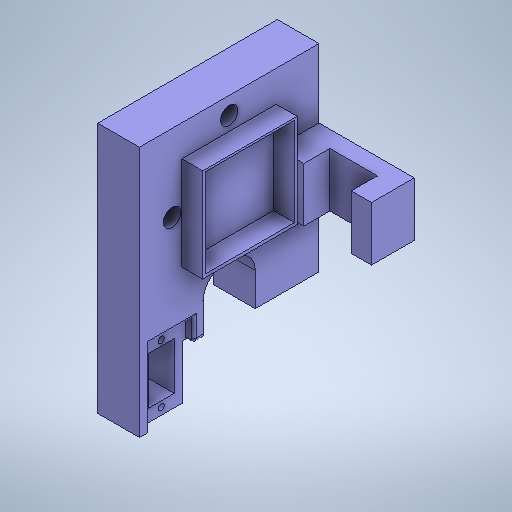
# Autodesk Inventor part: HolderWStepper
Saved by Autodesk Inventor 2025.1 (Build 291241000, 241)
## iProperties
Created: 2024-10-19
Part Number: HolderWStepper
Material: Generic
Document SubType Name: Modeling
Designer: 13156
Density: 1 g/cm^3
Appearance: Default
Author: 13156
Autodesk Inventor part; units mm, degrees
ref_plane "YZ Plane" through (0, 0, 0) normal (1, 0, 0) x (0, 1, 0)
ref_plane "XZ Plane" through (0, 0, 0) normal (0, 1, 0) x (-1, 0, 0)
ref_plane "XY Plane" through (0, 0, 0) normal (0, 0, 1) x (1, 0, 0)
sketch "Sketch1" plane through (0, 0, 0) normal (1, 0, 0) x (0, 1, 0)
  line L0 (-4.3, 12.5) -> (-12.5, 12.5)
  line L1 (-4.3, -12.5) -> (-12.5, -12.5)
  line L2 (-12.5, 12.5) -> (-12.5, 18.5)
  line L3 (-12.5, 18.5) -> (23.4392, 18.5)
  line L4 (23.4392, 18.5) -> (23.4392, -18.5)
  line L5 (23.4392, -18.5) -> (-12.5, -18.5)
  line L6 (-12.5, -18.5) -> (-12.5, -12.5)
  line L7 (23.4392, 0) -> (13.4392, 0) construction
  line L8 (13.4392, 0) -> (0, 0) construction
  line L9 (10.7392, -7.25) -> (10.7392, 0) construction
  line L10 (10.7392, 0) -> (10.7392, 7.25) construction
  line L11 (-4.3, 12.5) -> (13.4392, 12.5)
  line L12 (13.4392, 12.5) -> (13.4392, -12.5)
  line L13 (13.4392, -12.5) -> (-4.3, -12.5)
  point P0 (-8.4, 12.5)
  dimension "d0" = 8.2
  dimension "d1" = 25
  dimension "d2" = 12.5
  dimension "d7" = 8.2
  dimension "d8" = 12.5
  dimension "d9" = 12.5
  dimension "d14" = 6
  dimension "d15" = 6
  dimension "d16" = 37
  dimension "d29" = 10
  dimension "d88" = 2.7
  dimension "d90" = 14.5
  dimension "d91" = 23.4392
  dimension "d92" = 15.0392
  constraints: 28 end point, 5 perpendicular, 4 horizontal, 3 point on line, 2 midpoint, 1 collinear, 1 vertical
  measures "d0" distance of L0.start L0.end
  measures "d1" distance between parallel lines of L1 L0
  measures "d2" vertical distance of point (-8.4, 12.5) L8.end
  measures "d7" distance of L1.start L1.end
  measures "d8" vertical distance of L1.start L8.end
  measures "d9" horizontal distance of L1.end L8.end
  measures "d14" distance of L0.end L2.end
  measures "d15" distance of L5.end L1.end
  measures "d16" distance of L3.end L4.end
  measures "d29" distance of L7.start L7.end
  measures "d88" distance from line of L9 L7.end
  measures "d90" distance of L10.end L9.start
  measures "d91" distance of L7.start L8.end
  measures "d92" horizontal distance of L1.start L9.start
extrude "Extrusion1" add sketch "Sketch1" along normal blind 20
sketch "Sketch2" plane through (0, 23.4392, 18.5) normal (0, 1, 0) x (1, 0, 0)
  line L0 (0, 31) -> (0, 37) projected
  line L1 (0, 37) -> (70, 37)
  line L2 (70, 37) -> (70, 0.0995)
  line L3 (70, 0.0995) -> (0, 0.0995)
  line L4 (0, 0.0995) -> (0, 37)
  line L5 (20, 37) -> (20, 0) projected
  point P0 (0, 18.5)
  point P1 (70, 18.5498)
  dimension "d19" = 50
  constraints: 8 end point, 2 parallel, 1 horizontal, 1 midpoint, 1 perpendicular
  measures "d19" distance from line of L5 point (70, 18.55)
extrude "Extrusion2" add sketch "Sketch2" along normal blind 10
sketch "Sketch3" plane through (0, 23.4392, 18.5) normal (0, -1, 0) x (1, 0, 0)
  line L0 (110.5, -8.5498) -> (110.5, -28.5498)
  line L1 (110.5, -28.5498) -> (70, -28.5498)
  line L2 (70, -28.5498) -> (70, -8.5498)
  line L3 (70, -0.0995) -> (70, -37) projected
  line L4 (110.5, -8.5498) -> (119.5, -8.5498)
  line L5 (119.5, -8.5498) -> (119.5, -37)
  line L6 (119.5, -37) -> (70, -37)
  line L7 (70, -37) -> (0, -37) projected
  line L8 (70, -37) -> (59, -37)
  line L9 (59, -37) -> (59, -8.5498)
  line L10 (59, -8.5498) -> (70, -8.5498)
  point P0 (0, -18.5)
  point P1 (70, -18.5498)
  point P2 (70, -18.5498)
  point P3 (110.5, -18.5498)
  dimension "d22" = 20
  dimension "d23" = 20
  dimension "d24" = 0
  dimension "d25" = 40.5
  dimension "d26" = 9
  dimension "d30" = 11
  constraints: 18 end point, 4 perpendicular, 3 midpoint, 2 point on line, 2 vertical, 1 horizontal
  measures "d22" distance of L0.start L0.end
  measures "d23" distance of L1.end L2.end
  measures "d24" distance of point (70, -18.55) point (70, -18.55)
  measures "d25" distance from line of L2 point (110.5, -18.55)
  measures "d26" distance between parallel lines of L0 L5
  measures "d30" distance between parallel lines of L9 L2
extrude "Extrusion3" add sketch "Sketch3" along normal blind 9.5 and the other way blind 10
sketch "Sketch4" plane through (0, 33.4392, 18.5) normal (0, 1, 0) x (1, 0, 0)
  line L0 (110.5, 8.5498) -> (119.5, 8.5498) projected
  line L1 (62.5, 28.5653) -> (119.5, 28.5653)
  line L2 (119.5, 28.5653) -> (119.5, 8.5498)
  line L3 (119.5, 8.5498) -> (62.5, 8.5498)
  line L4 (62.5, 8.5498) -> (62.5, 28.5653)
  line L5 (70, 0.0995) -> (70, 28.5498) projected
  line L6 (110.5, 28.5498) -> (110.5, 8.5498) projected
  point P0 (0, 18.5)
  point P1 (70, 14.3246)
  point P2 (110.5, 8.5498)
  dimension "d33" = 7.5
  dimension "d34" = 9
  constraints: 8 end point, 2 parallel, 1 horizontal, 1 midpoint, 1 perpendicular, 1 point on line
  measures "d33" distance from line of point (70, 14.325) L4
  measures "d34" distance between parallel lines of L6 L2
extrude "Extrusion4" cut sketch "Sketch4" against normal blind 14.2625
sketch "Sketch5" plane through (0, 33.4392, 18.5) normal (0, 1, 0) x (1, 0, 0)
  line L0 (62.5, 8.5498) -> (62.5, 28.5653) projected
  line L1 (62.5, 8.5498) -> (70, 8.5498)
  line L2 (70, 8.5498) -> (70, -1.0168)
  line L3 (70, -1.0168) -> (62.5, -1.0168)
  line L4 (62.5, -1.0168) -> (62.5, 8.5498)
  line L5 (70, 0.0995) -> (70, 8.5498) projected
  point P0 (0, 18.5)
  dimension "d47" = 0
  constraints: 8 end point, 2 parallel, 1 horizontal, 1 perpendicular
  measures "d47" distance between parallel lines of L2 L5
extrude "Extrusion5" cut sketch "Sketch5" against normal blind 14.2625
sketch "Sketch7" plane through (59, 13.9392, 9.9502) normal (0, 0, 1) x (1, 0, 0)
  line L0 (3.5, 5.2375) -> (3.5, 9.5) projected
  line L1 (11, 0) -> (11, 5.2375) projected
  line L2 (3.5, 5.2375) -> (11, 5.2375)
  line L3 (11, 5.2375) -> (11, 0)
  line L4 (11, 0) -> (0, 0)
  line L5 (0, 0) -> (0, 9.5)
  line L6 (0, 9.5) -> (3.5, 9.5)
  line L7 (-39, 9.5) -> (3.5, 9.5) projected
  line L8 (3.5, 9.5) -> (3.5, 19.5) projected
  point P0 (-59, -13.9392)
  dimension "d42" = 11
  dimension "d43" = 0
  dimension "d44" = 0
  constraints: 10 end point, 3 perpendicular, 1 collinear, 1 horizontal
  measures "d42" distance of L1.start L4.end
  measures "d43" distance between parallel lines of L7 L6
  measures "d44" distance from line of L8 L6.end
extrude "Extrusion7" add sketch "Sketch7" along normal blind 8.45
sketch "Sketch8" plane through (62.5, 33.4392, 18.4005) normal (1, 0, 0) x (0, 0, -1)
  line L0 (28.4658, 0) -> (28.4658, -14.2625) projected
  line L1 (36.9005, 0) -> (0, 0) projected
  line L2 (28.4658, -9.8625) -> (0, -9.8625)
  line L3 (0, -9.8625) -> (0, 0)
  line L4 (0, 0) -> (28.4658, 0)
  line L5 (28.4658, 0) -> (28.4658, -9.8625)
  line L6 (28.4658, -14.2625) -> (8.4502, -14.2625) projected
  line L7 (8.4502, -14.2625) -> (8.4502, -19.5) projected
  line L8 (0, -10) -> (0, 0) projected
  point P0 (18.4005, -33.4392)
  dimension "d48" = 4.4
  dimension "d52" = 0
  constraints: 8 end point, 2 parallel, 2 point on line, 1 horizontal, 1 perpendicular
  measures "d48" distance between parallel lines of L2 L6
  measures "d52" distance between parallel lines of L8 L3
extrude "Extrusion8" add sketch "Sketch8" along normal blind 7.5
sketch "Sketch9" plane through (0, 33.4392, 18.5) normal (0, 1, 0) x (1, 0, 0)
  line L0 (59, 37) -> (59, 0.0998) projected
  line L1 (59, 0.0998) -> (59, 37)
  line L2 (119.5, 37) -> (119.5, 8.5498) projected
  line L3 (59, 37) -> (119.5, 37)
  line L4 (70, 28.5653) -> (119.5, 28.5653) projected
  line L5 (119.5, 37) -> (119.5, 28.5653)
  line L6 (119.5, 28.5653) -> (70, 28.5653)
  line L7 (0, 0.0995) -> (70, 0.0995) projected
  line L8 (70, 28.5653) -> (70, 0.0995)
  line L9 (70, 0.0995) -> (59, 0.0998)
  point P0 (0, 18.5)
  constraints: 12 end point, 3 perpendicular, 2 collinear
extrude "Extrusion9" add sketch "Sketch9" along normal blind 16
sketch "Sketch10" plane through (0, 33.4392, 18.5) normal (0, 1, 0) x (1, 0, 0)
  line L0 (59, 0.0998) -> (59, 37) projected
  line L1 (0, 0.0995) -> (70, 0.0995) projected
  line L2 (59, 37) -> (0, 37)
  line L3 (0, 37) -> (0, 0.0995)
  line L4 (0, 0.0995) -> (59, 0.0995)
  line L5 (59, 0.0995) -> (59, 37)
  point P0 (0, 18.5)
  point P1 (59, 0.0995)
  point P2 (59, 0.0998)
  constraints: 8 end point, 2 parallel, 1 horizontal, 1 perpendicular
extrude "Extrusion10" add sketch "Sketch10" along normal blind 16
sketch "Sketch12" plane through (0, 49.4392, 18.5) normal (0, 1, 0) x (1, 0, 0)
  line L0 (70, 28.5498) -> (70, 0.0998) projected
  line L1 (70, 0.0998) -> (-11.6844, 0.0998)
  line L2 (-11.6844, 0.0998) -> (-11.6844, -16.6848)
  line L3 (-11.6844, -16.6848) -> (70, -16.6848)
  line L4 (70, -16.6848) -> (70, 0.0998)
  point P0 (0, 18.5)
  constraints: 8 end point, 2 parallel, 1 horizontal, 1 perpendicular
extrude "Extrusion11" cut sketch "Sketch12" against normal blind 76.325
sketch "Sketch13" plane through (0, 19.1767, 18.5) normal (0, 1, 0) x (1, 0, 0)
  line L0 (110.5, 8.5498) -> (110.5, 28.5498) projected
  line L1 (70, 0.0998) -> (70, 28.5653) projected
  line L2 (110.5, 28.5498) -> (70, 28.5498)
  line L3 (70, 28.5498) -> (70, 28.5653)
  line L4 (70, 28.5653) -> (110.5, 28.5653)
  line L5 (110.5, 28.5653) -> (110.5, 28.5498)
  point P0 (0, 18.5)
  constraints: 8 end point, 2 parallel, 1 horizontal, 1 perpendicular
extrude "Extrusion12" cut sketch "Sketch13" against normal blind 76.325
sketch "Sketch14" plane through (0, 13.9392, 18.5) normal (0, -1, 0) x (1, 0, 0)
  circle A0 centre (114.7, -23.3) radius 2.1
  circle A1 centre (114.7, -13.2) radius 2.1
  line L0 (110.5, -8.5498) -> (110.5, -28.5653) projected
  line L1 (20, -11.25) -> (20, -25.75) projected
  point P0 (0, -18.5)
  point P1 (20, -18.5)
  dimension "d61" = 4.2
  dimension "d62" = 4.2
  dimension "d63" = 10.1
  dimension "d64" = 4.2
  dimension "d65" = 0
  dimension "d66" = 4.8
  constraints: 2 centre point, 1 midpoint
  measures "d61" diameter of A0
  measures "d62" diameter of A1
  measures "d63" distance of A0.centre A1.centre
  measures "d64" distance from line of L0 A0.centre
  measures "d65" horizontal distance of A0.centre A1.centre
  measures "d66" vertical distance of point (20, -18.5) A0.centre
extrude "Extrusion13" cut sketch "Sketch14" against normal blind 12.825
pattern_linear "Rectangular Pattern1" count 2 spacing 49 along (-1, 0, 0) of "Extrusion13"
sketch "Sketch15" plane through (0, 13.9392, 18.5) normal (0, -1, 0) x (1, 0, 0)
  line L0 (70, -0.0998) -> (70, -28.5653) projected
  line L1 (70, -0.0998) -> (119.5, -0.0998)
  line L2 (119.5, -0.0998) -> (119.5, -8.5498)
  line L3 (119.5, -8.5498) -> (110.5, -8.5498) projected
  line L4 (119.5, -8.5498) -> (110.5, -8.5498)
  line L5 (110.5, -8.5498) -> (68.2571, -8.5498)
  line L6 (68.2571, -8.5498) -> (59, -8.5498)
  line L7 (59, -37) -> (59, -0.0998) projected
  line L8 (59, -0.0998) -> (59, -8.5498)
  line L9 (59, -0.0998) -> (70, -0.0998)
  point P0 (0, -18.5)
  constraints: 14 end point, 4 point on line, 3 perpendicular, 1 collinear, 1 horizontal
extrude "Extrusion14" add sketch "Sketch15" against normal blind 35.5
sketch "Sketch16" plane through (119.5, 13.9392, 18.4002) normal (1, 0, 0) x (0, 0, -1)
  line L0 (7.45, 5.2375) -> (29.4655, 5.2375)
  line L1 (29.4655, 5.2375) -> (29.4655, 38.0522)
  line L2 (29.4655, 38.0522) -> (7.45, 38.0522)
  line L3 (7.45, 38.0522) -> (7.45, 5.2375)
  line L4 (28.4655, 5.2375) -> (8.45, 5.2375) projected
  line L5 (8.45, 5.2375) -> (8.45, 35.5) projected
  line L6 (28.4655, 35.5) -> (28.4655, 5.2375) projected
  point P0 (18.4002, -13.9392)
  dimension "d74" = 0
  dimension "d75" = 1
  dimension "d76" = 1
  constraints: 8 end point, 2 parallel, 1 horizontal, 1 perpendicular
  measures "d74" distance between parallel lines of L4 L0
  measures "d75" distance between parallel lines of L5 L3
  measures "d76" distance between parallel lines of L6 L1
extrude "Extrusion15" cut sketch "Sketch16" against normal blind 49.6875
sketch "Sketch19" plane through (0, 13.9392, 18.5) normal (0, -1, 0) x (1, 0, 0)
  line L0 (134.9623, 3.6486) -> (95.7961, 3.6486)
  line L1 (95.7961, 3.6486) -> (95.7961, -43.9762)
  line L2 (95.7961, -43.9762) -> (134.9623, -43.9762)
  line L3 (134.9623, -43.9762) -> (134.9623, 3.6486)
  point P0 (0, -18.5)
  constraints: 8 end point, 2 parallel, 1 horizontal, 1 perpendicular
extrude "Extrusion18" cut sketch "Sketch19" against normal blind 65.5625
sketch "Sketch20" plane through (0, 49.4392, 18.5) normal (0, 1, 0) x (1, 0, 0)
  line L0 (95.7961, 28.5653) -> (95.7961, 29.5653) projected
  line L1 (95.7961, 7.5498) -> (69.8125, 7.5498) projected
  line L2 (95.7961, 29.5653) -> (69.8125, 29.5653)
  line L3 (69.8125, 29.5653) -> (69.8125, 7.5498)
  line L4 (69.8125, 7.5498) -> (95.7961, 7.5498)
  line L5 (95.7961, 7.5498) -> (95.7961, 29.5653)
  point P0 (0, 18.5)
  point P1 (95.7961, 7.5498)
  constraints: 8 end point, 2 parallel, 1 horizontal, 1 perpendicular
extrude "Extrusion19" cut sketch "Sketch20" against normal blind 65.5625
sketch "Sketch22" plane through (20, 0, 0) normal (1, 0, 0) x (0, 0, -1)
  line L0 (-18.4002, -12.5) -> (-18.4002, 49.4392) projected
  line L1 (-18.4002, 49.4392) -> (-38.4002, 49.4392)
  line L2 (-38.4002, 49.4392) -> (-38.4002, -38.25)
  line L3 (-38.4002, -38.25) -> (-18.4002, -38.25)
  line L4 (-18.4002, -38.25) -> (-18.4002, 49.4392)
  line L5 (-18.4002, -12.5) -> (-12.5, -12.5) projected
  point P0 (0, 0)
  point P1 (-15.4501, -12.5)
  dimension "d104" = 20
  dimension "d107" = 25.75
  constraints: 8 end point, 2 parallel, 1 horizontal, 1 midpoint, 1 perpendicular
  measures "d104" distance of L2.end L3.end
  measures "d107" distance from line of point (-15.45, -12.5) L3
extrude "Extrusion21" add sketch "Sketch22" against normal blind 20
sketch "Sketch23" plane through (20, 0, 0) normal (1, 0, 0) x (0, 0, -1)
  line L0 (-34.9002, -9.45) -> (-22.4002, -9.45)
  line L1 (-22.4002, -9.45) -> (-22.4002, -32.25)
  line L2 (-22.4002, -32.25) -> (-34.9002, -32.25)
  line L3 (-34.9002, -32.25) -> (-34.9002, -9.45)
  line L4 (-18.4002, -38.25) -> (-18.4002, -12.5) projected
  line L5 (-38.4002, -38.25) -> (-18.4002, -38.25) projected
  point P0 (0, 0)
  dimension "d100" = 22.8
  dimension "d101" = 12.5
  dimension "d102" = 4
  dimension "d103" = 6
  constraints: 8 end point, 2 parallel, 1 horizontal, 1 perpendicular
  measures "d100" distance of L2.end L0.start
  measures "d101" distance of L0.start L0.end
  measures "d102" distance between parallel lines of L4 L1
  measures "d103" distance between parallel lines of L5 L2
extrude "Extrusion22" cut sketch "Sketch23" against normal blind 29.2125
sketch "Sketch24" plane through (0, 23.4392, 18.5) normal (0, -1, 0) x (1, 0, 0)
  line L0 (20, -31) -> (20, -37) projected
  line L1 (59, -37) -> (95.7961, -37) projected
  line L2 (65.7176, -37) -> (26.1847, -37)
  line L3 (26.1847, -37) -> (26.1847, -61.5946)
  line L4 (26.1847, -61.5946) -> (65.7176, -61.5946)
  line L5 (65.7176, -61.5946) -> (65.7176, -37)
  point P0 (0, -18.5)
  point P1 (20, -34)
  constraints: 8 end point, 2 parallel, 1 horizontal, 1 midpoint, 1 perpendicular, 1 point on line
extrude "Extrusion23" add sketch "Sketch24" against normal blind 26.35
sketch "Sketch25" plane through (0, 49.7892, 18.5) normal (0, 1, 0) x (1, 0, 0)
  line L0 (56, 53.5946) -> (33.24, 53.5946)
  line L1 (33.24, 53.5946) -> (33.24, 41.0946)
  line L2 (33.24, 41.0946) -> (56, 41.0946)
  line L3 (56, 41.0946) -> (56, 53.5946)
  line L4 (59, 37) -> (59, 0.0998) projected
  line L5 (26.1847, 61.5946) -> (65.7176, 61.5946) projected
  point P0 (0, 18.5)
  point P1 (20, -37)
  point P2 (44.62, 53.5946)
  point P3 (56, 47.3446)
  dimension "d112" = 22.76
  dimension "d113" = 12.5
  dimension "d115" = 3
  dimension "d118" = 8
  constraints: 8 end point, 2 midpoint, 2 parallel, 1 horizontal, 1 perpendicular
  measures "d112" distance between parallel lines of L1 L3
  measures "d113" distance between parallel lines of L2 L0
  measures "d115" distance from line of L4 point (56, 47.345)
  measures "d118" distance between parallel lines of L5 L0
extrude "Extrusion24" cut sketch "Sketch25" along normal mid plane 71.9725
sketch "Sketch27" plane through (26.1847, 23.4392, -43.0946) normal (-1, 0, 0) x (0, 0, 1)
  line L0 (0, 0) -> (24.5946, 0) projected
  line L1 (0, 0) -> (24.5946, 0)
  line L2 (24.5946, 0) -> (24.5946, 26.0294)
  line L3 (24.5946, 26.0294) -> (0, 26.0294)
  line L4 (0, 26.0294) -> (0, 0)
  point P0 (43.0946, -23.4392)
  point P1 (24.5946, 0)
  constraints: 8 end point, 2 parallel, 1 horizontal, 1 perpendicular
extrude "Extrusion25" add sketch "Sketch27" along normal up to surface (26.1847 mm away)
sketch "Sketch28" plane through (0, 0, 0) normal (-1, 0, 0) x (0, 0, 1)
  line L0 (-11.0653, 49.4392) -> (-18.5, 49.4392) projected
  line L1 (-18.5, 49.4392) -> (-46.1884, 49.4392)
  line L2 (-46.1884, 49.4392) -> (-46.1884, 57.0706)
  line L3 (-46.1884, 57.0706) -> (-18.5, 57.0706)
  line L4 (-18.5, 57.0706) -> (-18.5, 49.4392)
  point P0 (0, 0)
  constraints: 8 end point, 2 parallel, 1 horizontal, 1 perpendicular
extrude "Extrusion26" cut sketch "Sketch28" against normal blind 84.6125
sketch "Sketch29" plane through (20, 0, 0) normal (1, 0, 0) x (0, 0, -1)
  line L0 (18.5, -12.5) -> (18.5, 23.4392) projected
  line L1 (43.0946, 23.4392) -> (18.5, 23.4392) projected
  line L2 (18.5, -12.5) -> (43.0946, -12.5)
  line L3 (43.0946, -12.5) -> (43.0946, 23.4392)
  line L4 (43.0946, 23.4392) -> (18.5, 23.4392)
  line L5 (18.5, 23.4392) -> (18.5, -12.5)
  point P0 (0, 0)
  constraints: 8 end point, 2 parallel, 1 horizontal, 1 perpendicular
extrude "Extrusion27" add sketch "Sketch29" against normal up to surface (20 mm away)
sketch "Sketch31" plane through (0, -38.25, 38.4002) normal (0, -1, 0) x (1, 0, 0)
  line L0 (20, -21.5) -> (0, -21.5) projected
  line L1 (29.0845, 0.2184) -> (16, 0.2184)
  line L2 (16, 0.2184) -> (16, -21.5)
  line L3 (16, -21.5) -> (29.0845, -21.5)
  line L4 (29.0845, -21.5) -> (29.0845, 0.2184)
  line L5 (20, 0) -> (20, -21.5) projected
  point P0 (0, -38.4002)
  dimension "d147" = 4
  constraints: 8 end point, 2 parallel, 1 horizontal, 1 perpendicular, 1 point on line
  measures "d147" distance between parallel lines of L2 L5
extrude "Extrusion29" cut sketch "Sketch31" against normal blind 36.9875
fillet "Fillet3" radius 2 2 edges at (20, -12.5, 14.7001) (0, -12.5, 15.4501) curvature continuous yes
fillet "Fillet6" radius 10 2 edges at (10, 13.4392, 12.5) (10, 13.4392, -12.5)
sketch "Sketch34" plane through (0, 23.4392, 18.5) normal (0, -1, 0) x (1, 0, 0)
  circle A0 centre (58.6, -47.3446) radius 1.5
  line L0 (56, -41.0946) -> (56, -53.5946) projected
  line L1 (33.24, -41.0946) -> (56, -41.0946) projected
  circle A1 centre (30.64, -47.3446) radius 1.5
  line L2 (33.24, -53.5946) -> (33.24, -41.0946) projected
  line L3 (56, -53.5946) -> (33.24, -53.5946) projected
  point P0 (0, -18.5)
  dimension "d156" = 3
  dimension "d157" = 2.6
  dimension "d160" = 6.25
  dimension "d161" = 2.6
  dimension "d162" = 6.25
  constraints: 2 centre point, 1 equal radius
  measures "d156" diameter of A0
  measures "d157" distance from line of L0 A0.centre
  measures "d160" distance from line of L1 A0.centre
  measures "d161" distance from line of L2 A1.centre
  measures "d162" distance from line of L3 A1.centre
extrude "Extrusion30" cut sketch "Sketch34" against normal blind 6 contours A0 | A1
ref_plane "Work Plane1" through (16, -1.2625, 36.4002) normal (1, 0, 0) x (0, 0, -1)
sketch "Sketch36" plane through (16, -1.2625, 36.4002) normal (1, 0, 0) x (0, 0, -1)
  circle A0 centre (7.75, -33.5875) radius 1.5
  line L0 (1.5, -30.9875) -> (14, -30.9875) projected
  line L1 (1.5, -8.1875) -> (1.5, -30.9875) projected
  point P0 (36.4002, 1.2625)
  point P1 (7.75, -30.9875)
  dimension "d169" = 3
  dimension "d170" = 2.6
  dimension "d171" = 6.25
  constraints: 1 centre point, 1 midpoint
  measures "d169" diameter of A0
  measures "d170" distance of point (7.75, -30.987) A0.centre
  measures "d171" distance from line of L1 A0.centre
ref_plane "Work Plane2" through (16, -1.2625, 36.4002) normal (1, 0, 0) x (0, 0, -1)
sketch "Sketch35" plane through (16, -1.2625, 36.4002) normal (1, 0, 0) x (0, 0, -1)
  circle A0 centre (7.75, -5.5875) radius 1.5
  line L0 (14, -30.9875) -> (14, -8.1875) projected
  line L1 (14, -8.1875) -> (1.5, -8.1875) projected
  point P0 (36.4002, 1.2625)
  dimension "d164" = 3
  dimension "d165" = 6.25
  dimension "d166" = 2.6
  constraints: 1 centre point
  measures "d164" diameter of A0
  measures "d165" distance from line of L0 A0.centre
  measures "d166" distance from line of L1 A0.centre
extrude "Extrusion31" cut sketch "Sketch35" against normal blind 6
extrude "Extrusion32" cut sketch "Sketch36" against normal blind 6
sketch "Sketch37" plane through (20, 0, 0) normal (1, 0, 0) x (0, 0, -1)
  line L0 (-38.4002, 49.4392) -> (-38.4002, -1.2625) projected
  line L1 (-38.4002, 49.4392) -> (-43.0952, 49.4392)
  line L2 (-43.0952, 49.4392) -> (-43.0952, -38.25)
  line L3 (-43.0952, -38.25) -> (-38.4002, -38.25)
  line L4 (-38.4002, -38.25) -> (-38.4002, 49.4392)
  point P0 (0, 0)
  dimension "d174" = 4.695
  constraints: 8 end point, 2 parallel, 1 horizontal, 1 perpendicular
  measures "d174" distance of L0.start L1.end
extrude "Extrusion33" add sketch "Sketch37" against normal up to surface (20 mm away)
fillet "Fillet10" radius 1 2 edges at (18, -38.25, 38.4002) (20, -19.7563, 38.4002)
fillet "Fillet11" radius 1 6 edges at (16, -1.2625, 27.6502) (20, -1.2625, 38.9002) (20, -1.2625, 27.6502) (19.4819, -11.9822, 16.9002) (17, -12.5, 16.9002) (20, -5.8813, 16.9002)
sketch "Sketch38" plane through (0, 13.9392, 18.5) normal (0, -1, 0) x (1, 0, 0)
  line L0 (20, 0.9002) -> (20, -59.5946) projected
  line L1 (104.7813, 12.4514) -> (20, 12.4514)
  line L2 (20, 12.4514) -> (20, -41.0946)
  line L3 (20, -41.0946) -> (104.7813, -41.0946)
  line L4 (104.7813, -41.0946) -> (104.7813, 12.4514)
  line L5 (33.24, -41.0946) -> (56, -41.0946) projected
  point P0 (0, -18.5)
  dimension "d181" = 0
  dimension "d182" = 53.546
  constraints: 8 end point, 2 parallel, 1 horizontal, 1 perpendicular, 1 point on line
  measures "d181" distance between parallel lines of L5 L3
  measures "d182" distance between parallel lines of L1 L3
extrude "Extrusion34" cut sketch "Sketch38" against normal blind 68.7375
sketch "Sketch39" plane through (20, 0, 0) normal (1, 0, 0) x (0, 0, -1)
  line L0 (-43.0952, 47.4392) -> (-43.0952, -36.25) projected
  line L1 (-43.0952, 47.4392) -> (43.0946, 47.4392)
  line L2 (43.0946, 47.4392) -> (43.0946, 67.4392)
  line L3 (43.0946, 67.4392) -> (-43.0952, 67.4392)
  line L4 (-43.0952, 67.4392) -> (-43.0952, 47.4392)
  line L5 (43.0946, 25.4392) -> (43.0946, 47.4392) projected
  point P0 (0, 0)
  dimension "d185" = 20
  constraints: 8 end point, 2 parallel, 1 collinear, 1 horizontal, 1 perpendicular
  measures "d185" distance between parallel lines of L3 L1
extrude "Extrusion35" add sketch "Sketch39" against normal up to surface (20 mm away)
sketch "Sketch41" plane through (20, 0, 0) normal (1, 0, 0) x (0, 0, -1)
  line L0 (22.5946, 23.4392) -> (22.5946, 49.4392) projected
  line L1 (-43.0952, 67.4392) -> (43.0946, 67.4392) projected
  line L2 (-21.4054, 67.4392) -> (24.0946, 67.4392)
  line L3 (-21.25, 66.4392) -> (21.25, 66.4392)
  line L4 (21.25, 66.4392) -> (21.25, 23.9392)
  line L5 (21.25, 23.9392) -> (-21.25, 23.9392)
  line L6 (-21.25, 23.9392) -> (-21.25, 66.4392)
  line L7 (-22.75, 67.4392) -> (22.5946, 67.4392)
  line L8 (22.5946, 67.4392) -> (22.5946, 22.4392)
  line L9 (22.5946, 22.4392) -> (-22.75, 22.4392)
  line L10 (-22.75, 22.4392) -> (-22.75, 67.4392)
  point P0 (0, 0)
  dimension "d219" = 42.5
  dimension "d220" = 42.5
  dimension "d221" = 21.25
  dimension "d222" = 1
  dimension "d223" = 1.3446
  dimension "d224" = 1.5
  dimension "d225" = 1.5
  constraints: 18 end point, 4 parallel, 3 horizontal, 2 perpendicular, 2 point on line
  measures "d219" distance of L3.start L3.end
  measures "d220" distance of L5.end L3.start
  measures "d221" distance from line of point (0, 0) L4
  measures "d222" distance between parallel lines of L1 L3
  measures "d223" distance between parallel lines of L4 L8
  measures "d224" distance between parallel lines of L9 L5
  measures "d225" distance between parallel lines of L10 L6
extrude "Extrusion37" add sketch "Sketch41" along normal blind 10
sketch "Sketch40" plane through (20, 0, 0) normal (1, 0, 0) x (0, 0, -1)
  circle A0 centre (-27.4054, 45.4392) radius 4.2
  line L0 (22.5946, 49.4392) -> (22.5946, 23.4392) projected
  line L1 (43.0946, 67.4392) -> (-43.0952, 67.4392) projected
  point P0 (0, 0)
  point P1 (22.5946, 36.4392)
  dimension "d188" = 8.4
  dimension "d189" = 50
  dimension "d190" = 22
  constraints: 1 centre point, 1 midpoint
  measures "d188" diameter of A0
  measures "d189" horizontal distance of point (22.595, 36.439) A0.centre
  measures "d190" distance from line of L1 A0.centre
extrude "Extrusion36" cut sketch "Sketch40" against normal blind 6
sketch "Sketch42" plane through (20, 0, 0) normal (1, 0, 0) x (0, 0, -1)
  line L0 (-43.0952, 67.4392) -> (-43.0952, -38.25) projected
  line L1 (-43.0952, 67.4392) -> (43.0946, 67.4392)
  line L2 (43.0946, 67.4392) -> (43.0946, 82.4392)
  line L3 (43.0946, 82.4392) -> (-43.0952, 82.4392)
  line L4 (-43.0952, 82.4392) -> (-43.0952, 67.4392)
  line L5 (43.0946, 49.4392) -> (43.0946, 67.4392) projected
  point P0 (0, 0)
  point P1 (-0.0003, 67.4392)
  dimension "d200" = 0
  dimension "d201" = 15
  constraints: 8 end point, 2 parallel, 1 horizontal, 1 midpoint, 1 perpendicular
  measures "d200" distance between parallel lines of L5 L2
  measures "d201" distance from line of point (0, 67.439) L3
extrude "Extrusion38" add sketch "Sketch42" against normal up to surface (20 mm away)
sketch "Sketch43" plane through (20, 0, 0) normal (1, 0, 0) x (0, 0, -1)
  circle A0 centre (0, 74.0792) radius 4.2
  circle A1 centre (-27.4054, 45.4392) radius 4.2 projected
  line L0 (-19.9054, 23.4392) -> (-19.9054, 65.9392) projected
  line L1 (43.0946, 82.4392) -> (-43.0952, 82.4392) projected
  point P0 (0, 0)
  dimension "d211" = 19.9054
  dimension "d212" = 8.36
  constraints: 1 centre point, 1 equal radius
  measures "d211" distance from line of L0 A0.centre
  measures "d212" distance from line of L1 A0.centre
extrude "Extrusion39" cut sketch "Sketch43" against normal blind 8.4125 contours A0
body "Solid1"
